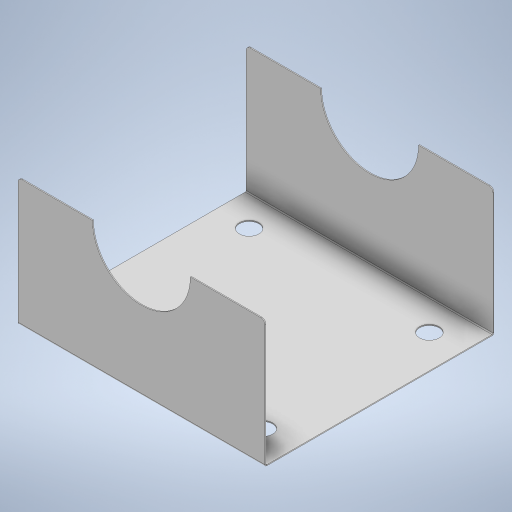
# Autodesk Inventor part: Крепление
Saved by Autodesk Inventor 2024.2 (Build 282272000, 272)
## iProperties
Created: 2024-04-09
Part Number: Крепление
Material: Generic
Document SubType Name: Sheet Metal
Designer: pokla
Density: 1 g/cm^3
Sheet Metal Rule: Default_mm
Appearance: Default
Author: pokla
Autodesk Inventor part; units mm, degrees
ref_plane "YZ Plane" through (0, 0, 0) normal (1, 0, 0) x (0, 1, 0)
ref_plane "XZ Plane" through (0, 0, 0) normal (0, 1, 0) x (-1, 0, 0)
ref_plane "XY Plane" through (0, 0, 0) normal (0, 0, 1) x (1, 0, 0)
sketch "Sketch4" plane through (0, 0, 0) normal (0, 1, 0) x (-1, 0, 0)
  line L0 (63, -57.5) -> (-63, -57.5)
  line L1 (-63, -57.5) -> (-63, 57.5)
  line L2 (-63, 57.5) -> (63, 57.5)
  line L3 (63, 57.5) -> (63, -57.5)
  line L4 (63, -57.5) -> (-63, 57.5) construction
  point P0 (0, 0)
  point P1 (0, 0)
  dimension "d24" = 126
  dimension "d25" = 115
  measures "d24" distance of L1.end L2.end
  measures "d25" distance of L0.end L1.end
extrude "Plate4" add sketch "Sketch4" along normal mid plane 0.5
sketch "Sketch5" plane through (63, 0.75, 58) normal (0, 0, 1) x (1, 0, 0)
  line L0 (-126, 0) -> (0, 0)
  line L1 (0, 0) -> (0, 64)
  line L2 (0, 64) -> (-126, 64)
  line L3 (-126, 64) -> (-126, 0)
  constraints: 6 end point, 1 horizontal, 1 perpendicular, 1 vertical
edge flange "Flange3" height 65 angle 90 thickness 0.5 bend radius 0.5 thickness toward (0, 0, 1) relief straight relief width 0.5 relief depth 0.25 corner gap 0.5 corner form 0 edges at (0, 0.25, 57.5) (0, 0.25, -57.5) wall of the first edge with corners at (-63, 0.75, 58) (63, 0.75, 58) (63, 64.75, 58) (-63, 64.75, 58)
bend "Bend3"
corner "Corner3"
sketch "Sketch6" plane through (-63, 64.75, 58.5) normal (0, 0, 1) x (1, 0, 0)
  line L0 (0, 0) -> (126, 0) projected
  circle A0 centre (63, 0) radius 25
  point P0 (63, -64.75)
  dimension "d37" = 50
  constraints: 1 centre point, 1 midpoint
  measures "d37" diameter of A0
extrude "Extrusion1" cut sketch "Sketch6" against normal through all
fillet "Fillet1" radius 2 4 edges at (63, 64.75, -58.25) (-63, 64.75, -58.25) (-63, 64.75, 58.25) (63, 64.75, 58.25)
sketch "Sketch7" plane through (0, -0.25, 0) normal (0, -1, 0) x (1, 0, 0)
  circle A0 centre (46, -42.5) radius 5
  line L0 (63, 57.5) -> (63, -57.5) projected
  line L1 (63, -57.5) -> (-63, -57.5) projected
  line L2 (25, 58) -> (-25, 58) construction
  line L3 (0, -74.3103) -> (0, 74.3103) construction
  line L4 (114.9724, 0) -> (-114.9724, 0) construction
  circle A1 centre (-46, -42.5) radius 5
  circle A2 centre (46, 42.5) radius 5
  circle A3 centre (-46, 42.5) radius 5
  point P0 (0, 0)
  point P1 (0, 0)
  dimension "d41" = 10
  dimension "d42" = 17
  dimension "d43" = 15
  constraints: 4 centre point, 4 end point, 3 symmetric about line, 2 midpoint, 1 coincident, 1 horizontal, 1 vertical, 3 other
  measures "d41" diameter of A0
  measures "d42" distance from line of L0 A0.centre
  measures "d43" distance from line of L1 A0.centre
extrude "Extrusion2" cut sketch "Sketch7" against normal up to surface (0.5 mm away)
equation "\"d26\" = Thickness"
equation "\"d27\" = BendReliefWidth"
equation "\"d28\" = BendReliefDepth"
equation "\"d29\" = MinimumRemnant"
equation "\"d30\" = TransitionRadius"
equation "\"d33\" = BendRadius"
equation "\"d34\" = CornerReliefSize"
equation "\"d35\" = GapSize"
equation "\"d36\" = JacobiRadiusSize"
equation "\"BendRadius\" = Thickness"
equation "\"BendReliefWidth\" = Thickness"
equation "\"BendReliefDepth\" = 0.5 * Thickness"
equation "\"CornerReliefSize\" = 4 * Thickness"
equation "\"MinimumRemnant\" = 2 * Thickness"
equation "\"TransitionRadius\" = BendRadius"
equation "\"JacobiRadiusSize\" = BendRadius"
equation "\"GapSize\" = Thickness"
equation "\"Thickness\" = 0.5"
body "Solid2"
